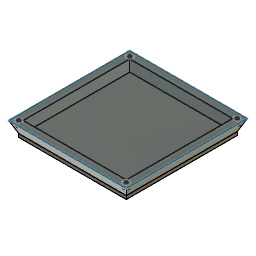
OmniSort (Autodesk Fusion 360 design; units mm, degrees)
Autodesk Fusion 360 part; units mm, degrees
note: some values were not read from the file. Set by a fixed rule: which sketch regions a step uses.
sketch "Sketch1" plane through (0, 0, 0) normal (0, 0, 1) x (1, 0, 0)
  line L0 (-132.8, 97) -> (-38, 97)
  line L1 (-38, 97) -> (-38, -0.8)
  line L2 (-38, -0.8) -> (-132.8, -0.8)
  line L3 (-132.8, -0.8) -> (-132.8, 97)
  line L4 (-132.8, 97) -> (-38, -0.8) construction
  line L5 (-38, 97) -> (-132.8, -0.8) construction
  point P0 (-85.4, 48.1)
  dimension "d3" = 94.8
  dimension "d4" = 97.8
  constraint horizontal L0
  constraint perpendicular L0 L1
  constraint parallel L0 L2
  constraint parallel L1 L3
  constraint coincident L4 P0
  constraint coincident L5 P0
  measures "d3" distance of L1.end L2.end
  measures "d4" distance of L0.end L1.end
extrude "Extrude1" add sketch "Sketch1" along normal blind 3
sketch "Sketch2" plane through (0, 0, 3) normal (0, 0, 1) x (-1, 0, 0)
  line L0 (132.8, 0.8) -> (38, 0.8)
  line L1 (38, 0.8) -> (38, -97)
  line L2 (38, -97) -> (132.8, -97)
  line L3 (132.8, -97) -> (132.8, 0.8)
  line L4 (130.8, -95) -> (40, -95)
  line L5 (40, -95) -> (40, -1.2)
  line L6 (40, -1.2) -> (130.8, -1.2)
  line L7 (130.8, -1.2) -> (130.8, -95)
  line L8 (130.8, -95) -> (40, -1.2) construction
  line L9 (40, -95) -> (130.8, -1.2) construction
  point P0 (85.4, -48.1)
  dimension "d7" = 90.8
  dimension "d8" = 93.8
  constraint horizontal L4
  constraint perpendicular L4 L5
  constraint parallel L4 L6
  constraint parallel L5 L7
  constraint coincident L8 P0
  constraint coincident L9 P0
  measures "d7" distance of L5.end L6.end
  measures "d8" distance of L4.end L5.end
extrude "Extrude2" add sketch "Sketch2" along normal blind 10
sketch "Sketch3" plane through (0, 0, 13) normal (0, 0, 1) x (-1, 0, 0)
  line L0 (40, -1.2) -> (130.8, -1.2)
  line L1 (130.8, -1.2) -> (130.8, -95)
  line L2 (130.8, -95) -> (40, -95)
  line L3 (40, -95) -> (40, -1.2)
  line L4 (132.8, -97) -> (132.8, 0.8)
  line L5 (132.8, 0.8) -> (38, 0.8)
  line L6 (38, 0.8) -> (38, -97)
  line L7 (38, -97) -> (132.8, -97)
  line L8 (33.5, 5.3) -> (33.5, -101.5)
  line L9 (33.5, -101.5) -> (137.3, -101.5)
  line L10 (137.3, -101.5) -> (137.3, 5.3)
  line L11 (137.3, 5.3) -> (33.5, 5.3)
  circle A0 centre (38, 0.8) radius 2.35
  circle A1 centre (38, -97) radius 2.35
  circle A2 centre (132.8, -97) radius 2.35
  circle A3 centre (132.8, 0.8) radius 2.35
  dimension "d21" = 4.7
  dimension "d22" = 4.7
  dimension "d23" = 4.7
  dimension "d24" = 4.7
  constraint coincident L5.end L6.start
  constraint coincident L6.end L7.start
  constraint coincident L4.start L7.end
  constraint coincident L4.end L5.start
  measures "d21" diameter of A0
  measures "d22" diameter of A1
  measures "d23" diameter of A2
  measures "d24" diameter of A3
extrude "Extrude3" add sketch "Sketch3" against normal blind 10 contours L4 L7 A2 | L4 L5 A3 | L6 L7 A1 | L5 L6 A0 | L8 L9 L10 L11 picked at (131.2421, -97.1167) picked at (132.1221, 2.2076) picked at (39.5582, -97.1149) picked at (38.0383, 2.362)
chamfer "Chamfer1" distance 4.5 distance2 10 4 edges at (-85.4, -5.3, 3) (-33.5, 48.1, 3) (-85.4, 101.5, 3) (-137.3, 48.1, 3) measured on face at (-35, 31.8, 3) measured on face at (-35, 31.8, 3) measured on face at (-35, 31.8, 3) measured on face at (-35, 31.8, 3)
extrude "Extrude4" cut sketch "Sketch3" against normal blind 4 contours L4 L7 A2 | L4 L7 A2 | L4 L5 A3 | L4 L5 A3 | L6 L7 A1 | L6 L7 A1 | L5 L6 A0 | L5 L6 A0
